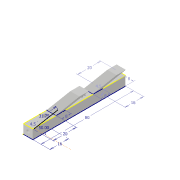
# Autodesk Inventor part: MineralStop1.25x50
Saved by Autodesk Inventor 2018 (Build 220112000, 112)
## iProperties
Created: 2018-12-12
Part Number: MineralStop1.25x50
Material: Generic
Document SubType Name: Modeling
Designer: ball
Density: 1 g/cm^3
Appearance: Default
Author: ball
Autodesk Inventor part; units mm, degrees
ref_plane "YZ Plane" through (0, 0, 0) normal (1, 0, 0) x (0, 1, 0)
ref_plane "XZ Plane" through (0, 0, 0) normal (0, 1, 0) x (-1, 0, 0)
ref_plane "XY Plane" through (0, 0, 0) normal (0, 0, 1) x (1, 0, 0)
sketch "Sketch1" plane through (0, 0, 0) normal (0, 1, 0) x (-1, 0, 0)
  line L0 (0, 0) -> (-8, 0)
  line L1 (-8, 0) -> (-8, -80)
  line L2 (-8, -80) -> (0, -80)
  line L3 (0, -80) -> (0, 0)
  circle A0 centre (-4, -16) radius 2.25
  circle A1 centre (-4, -64) radius 2.25
  dimension "d0" = 8
  dimension "d1" = 80
  dimension "d6" = 4.5
  dimension "d7" = 4.5
  dimension "d26" = 16
  dimension "d27" = 16
  constraints: 8 end point, 2 centre point, 2 parallel, 1 horizontal, 1 perpendicular
  measures "d0" distance of L2.end L1.end
  measures "d1" distance of L1.end L0.end
  measures "d6" diameter of A0
  measures "d7" diameter of A1
  measures "d26" distance from line of L0 A0.centre
  measures "d27" distance from line of L2 A1.centre
extrude "Extrusion1" [suppressed]
extrude "Extrusion2" add sketch "Sketch1" along normal blind 8
sketch "Sketch2" plane through (0, 0, 0) normal (0, 0, 1) x (1, 0, 0)
  circle A0 centre (4, 4) radius 1.35
  point P0 (0, 0)
  dimension "d10" = 2.7
  constraints: 1 centre point
  measures "d10" diameter of A0
hole "Hole1" at (4, 4, 0) direction (0, 0, -1) diameter 2.7 depth 10
sketch "Sketch3" plane through (8, 0, -80) normal (0, 0, -1) x (-1, 0, 0)
  circle A0 centre (4, 4) radius 1.35
  point P0 (8, 0)
  dimension "d18" = 2.7
  constraints: 1 centre point
  measures "d18" diameter of A0
hole "Hole2" at (4, 4, -80) direction (0, 0, 1) diameter 2.7 depth 10
sketch "Sketch5" plane through (0, 0, 0) normal (0, 0, 1) x (1, 0, 0)
  line L0 (9.3659, 8.9784) -> (29.7744, 33.3003)
  line L1 (9.3659, 8.9784) -> (41.1159, 8.9784) construction
  point P0 (0, 0)
  dimension "d33" = 31.75
  dimension "d34" = 50
  constraints: 4 end point, 1 equal length, 1 horizontal
  measures "d33" distance of L0.start L0.end
  measures "d34" angle of L1 L0
sketch "Sketch4" plane through (0, 8, 0) normal (0, 1, 0) x (1, 0, 0)
  line L0 (0, 80) -> (0, 0) projected
  line L1 (8, 0) -> (8, 80) projected
  line L2 (0, 28) -> (8, 28)
  line L3 (8, 28) -> (8, 20)
  line L4 (8, 20) -> (0, 20)
  line L5 (0, 20) -> (0, 28)
  line L6 (0, 0) -> (8, 0) projected
  line L7 (0, 60) -> (8, 60)
  line L8 (8, 60) -> (8, 52)
  line L9 (8, 52) -> (0, 52)
  line L10 (0, 52) -> (0, 60)
  line L11 (8, 80) -> (0, 80) projected
  line L12 (2.6299, 29.4213) -> (2.6299, 50.4758) construction
  line L13 (2.6299, 50.4758) -> (5.8779, 50.4758) construction
  line L14 (5.8779, 50.4758) -> (5.8779, 29.4213) construction
  line L15 (5.8779, 29.4213) -> (2.6299, 29.4213) construction
  line L16 (5.8137, 31.3702) -> (5.8137, 29.8832)
  line L17 (5.8137, 29.8832) -> (5.5025, 29.8832)
  line L18 (5.5025, 29.8832) -> (5.5025, 30.4365)
  line L19 (5.5025, 30.4365) -> (3.4598, 30.4365)
  line L20 (3.4598, 30.4365) -> (3.4598, 29.8832)
  line L21 (3.4598, 29.8832) -> (3.1807, 29.8832)
  spline S0 degree 2 poles (3.1807, 29.8832) (3.1807, 30.1969) (3.0028, 30.4933) (2.7558, 30.5131) knots 0 0 0 1 2 2 2
  line L22 (2.7558, 30.5131) -> (2.7558, 30.8292)
  line L23 (2.7558, 30.8292) -> (5.5025, 30.8292)
  line L24 (5.5025, 30.8292) -> (5.5025, 31.3702)
  line L25 (5.5025, 31.3702) -> (5.8137, 31.3702)
  line L26 (5.8137, 32.5854) -> (5.8137, 32.0964)
  line L27 (5.8137, 32.0964) -> (5.2308, 32.0964)
  line L28 (5.2308, 32.0964) -> (5.2308, 32.5854)
  line L29 (5.2308, 32.5854) -> (5.8137, 32.5854)
  line L30 (5.8137, 35.0801) -> (5.8137, 33.2005)
  line L31 (5.8137, 33.2005) -> (5.3815, 33.2005)
  spline S1 degree 2 poles (5.3815, 33.2005) (5.1913, 33.403) (4.838, 33.7636) (4.6479, 33.9365) knots 0 0 0 1 2 2 2
  spline S2 degree 2 poles (4.6479, 33.9365) (4.265, 34.2848) (3.8056, 34.5392) (3.561, 34.5392) knots 0 0 0 1 2 2 2
  spline S3 degree 2 poles (3.561, 34.5392) (3.4326, 34.5392) (3.2399, 34.4602) (3.1782, 34.3885) knots 0 0 0 1 2 2 2
  spline S4 degree 2 poles (3.1782, 34.3885) (3.1164, 34.3169) (3.0547, 34.1292) (3.0547, 34.0156) knots 0 0 0 1 2 2 2
  spline S5 degree 2 poles (3.0547, 34.0156) (3.0547, 33.9069) (3.109, 33.6846) (3.151, 33.5833) knots 0 0 0 1 2 2 2
  spline S6 degree 2 poles (3.151, 33.5833) (3.1856, 33.4969) (3.2844, 33.3363) (3.319, 33.2869) knots 0 0 0 1 2 2 2
  line L32 (3.319, 33.2869) -> (3.319, 33.2647)
  line L33 (3.319, 33.2647) -> (2.8843, 33.2647)
  spline S7 degree 2 poles (2.8843, 33.2647) (2.8225, 33.3907) (2.7015, 33.8427) (2.7015, 34.0452) knots 0 0 0 1 2 2 2
  spline S8 degree 2 poles (2.7015, 34.0452) (2.7015, 34.4725) (3.1535, 34.9542) (3.5388, 34.9542) knots 0 0 0 1 2 2 2
  spline S9 degree 2 poles (3.5388, 34.9542) (3.7191, 34.9542) (4.0205, 34.8702) (4.1489, 34.7961) knots 0 0 0 1 2 2 2
  spline S10 degree 2 poles (4.1489, 34.7961) (4.2823, 34.722) (4.5441, 34.5071) (4.6701, 34.3885) knots 0 0 0 1 2 2 2
  spline S11 degree 2 poles (4.6701, 34.3885) (4.88, 34.1959) (5.3296, 33.7241) (5.4605, 33.5833) knots 0 0 0 1 2 2 2
  line L34 (5.4605, 33.5833) -> (5.4605, 35.0801)
  line L35 (5.4605, 35.0801) -> (5.8137, 35.0801)
  spline S12 degree 2 poles (4.8455, 37.3353) (5.0653, 37.3353) (5.4407, 37.1945) (5.5791, 37.066) knots 0 0 0 1 2 2 2
  spline S13 degree 2 poles (5.5791, 37.066) (5.7174, 36.9376) (5.8779, 36.5547) (5.8779, 36.3176) knots 0 0 0 1 2 2 2
  spline S14 degree 2 poles (5.8779, 36.3176) (5.8779, 36.1003) (5.7816, 35.6754) (5.705, 35.5198) knots 0 0 0 1 2 2 2
  line L36 (5.705, 35.5198) -> (5.2728, 35.5198)
  line L37 (5.2728, 35.5198) -> (5.2728, 35.5494)
  spline S15 degree 2 poles (5.2728, 35.5494) (5.3074, 35.5964) (5.3963, 35.7717) (5.4358, 35.878) knots 0 0 0 1 2 2 2
  spline S16 degree 2 poles (5.4358, 35.878) (5.4778, 35.999) (5.5247, 36.1991) (5.5247, 36.325) knots 0 0 0 1 2 2 2
  spline S17 degree 2 poles (5.5247, 36.325) (5.5247, 36.4485) (5.4358, 36.6807) (5.3395, 36.7647) knots 0 0 0 1 2 2 2
  spline S18 degree 2 poles (5.3395, 36.7647) (5.2481, 36.8413) (5.006, 36.9203) (4.843, 36.9203) knots 0 0 0 1 2 2 2
  spline S19 degree 2 poles (4.843, 36.9203) (4.68, 36.9203) (4.4725, 36.8314) (4.4033, 36.7474) knots 0 0 0 1 2 2 2
  spline S20 degree 2 poles (4.4033, 36.7474) (4.3268, 36.661) (4.2625, 36.4041) (4.2625, 36.2485) knots 0 0 0 1 2 2 2
  spline S21 degree 2 poles (4.2625, 36.2485) (4.2625, 36.0805) (4.3144, 35.747) (4.3366, 35.6458) knots 0 0 0 1 2 2 2
  line L38 (4.3366, 35.6458) -> (2.7657, 35.6458)
  line L39 (2.7657, 35.6458) -> (2.7657, 37.318)
  line L40 (2.7657, 37.318) -> (3.1239, 37.318)
  line L41 (3.1239, 37.318) -> (3.1239, 36.0385)
  line L42 (3.1239, 36.0385) -> (3.9365, 36.0385)
  spline S22 degree 2 poles (3.9365, 36.0385) (3.9266, 36.1126) (3.9192, 36.2559) (3.9192, 36.3152) knots 0 0 0 1 2 2 2
  spline S23 degree 2 poles (3.9192, 36.3152) (3.9192, 36.5498) (3.9958, 36.8734) (4.1094, 37.0216) knots 0 0 0 1 2 2 2
  spline S24 degree 2 poles (4.1094, 37.0216) (4.223, 37.1722) (4.5688, 37.3353) (4.8455, 37.3353) knots 0 0 0 1 2 2 2
  line L43 (2.6299, 38.2319) -> (3.8155, 38.143)
  line L44 (3.8155, 38.143) -> (3.8155, 37.8737)
  line L45 (3.8155, 37.8737) -> (2.6299, 37.7848)
  line L46 (2.6299, 37.7848) -> (2.6299, 38.2319)
  line L47 (2.6299, 39.0025) -> (3.8155, 38.9136)
  line L48 (3.8155, 38.9136) -> (3.8155, 38.6444)
  line L49 (3.8155, 38.6444) -> (2.6299, 38.5555)
  line L50 (2.6299, 38.5555) -> (2.6299, 39.0025)
  line L51 (5.8137, 42.5989) -> (5.8137, 42.1271)
  line L52 (5.8137, 42.1271) -> (4.9541, 41.5713)
  line L53 (4.9541, 41.5713) -> (5.8137, 41.0008)
  line L54 (5.8137, 41.0008) -> (5.8137, 40.5636)
  line L55 (5.8137, 40.5636) -> (4.68, 41.3565)
  line L56 (4.68, 41.3565) -> (3.5265, 40.571)
  line L57 (3.5265, 40.571) -> (3.5265, 41.0428)
  line L58 (3.5265, 41.0428) -> (4.3786, 41.596)
  line L59 (4.3786, 41.596) -> (3.5265, 42.1617)
  line L60 (3.5265, 42.1617) -> (3.5265, 42.5989)
  line L61 (3.5265, 42.5989) -> (4.6553, 41.8109)
  line L62 (4.6553, 41.8109) -> (5.8137, 42.5989)
  spline S25 degree 2 poles (4.8455, 45.9976) (5.0653, 45.9976) (5.4407, 45.8568) (5.5791, 45.7284) knots 0 0 0 1 2 2 2
  spline S26 degree 2 poles (5.5791, 45.7284) (5.7174, 45.5999) (5.8779, 45.2171) (5.8779, 44.98) knots 0 0 0 1 2 2 2
  spline S27 degree 2 poles (5.8779, 44.98) (5.8779, 44.7626) (5.7816, 44.3378) (5.705, 44.1822) knots 0 0 0 1 2 2 2
  line L63 (5.705, 44.1822) -> (5.2728, 44.1822)
  line L64 (5.2728, 44.1822) -> (5.2728, 44.2118)
  spline S28 degree 2 poles (5.2728, 44.2118) (5.3074, 44.2587) (5.3963, 44.4341) (5.4358, 44.5403) knots 0 0 0 1 2 2 2
  spline S29 degree 2 poles (5.4358, 44.5403) (5.4778, 44.6613) (5.5247, 44.8614) (5.5247, 44.9874) knots 0 0 0 1 2 2 2
  spline S30 degree 2 poles (5.5247, 44.9874) (5.5247, 45.1109) (5.4358, 45.3431) (5.3395, 45.427) knots 0 0 0 1 2 2 2
  spline S31 degree 2 poles (5.3395, 45.427) (5.2481, 45.5036) (5.006, 45.5827) (4.843, 45.5827) knots 0 0 0 1 2 2 2
  spline S32 degree 2 poles (4.843, 45.5827) (4.68, 45.5827) (4.4725, 45.4937) (4.4033, 45.4098) knots 0 0 0 1 2 2 2
  spline S33 degree 2 poles (4.4033, 45.4098) (4.3268, 45.3233) (4.2625, 45.0664) (4.2625, 44.9108) knots 0 0 0 1 2 2 2
  spline S34 degree 2 poles (4.2625, 44.9108) (4.2625, 44.7428) (4.3144, 44.4094) (4.3366, 44.3081) knots 0 0 0 1 2 2 2
  line L65 (4.3366, 44.3081) -> (2.7657, 44.3081)
  line L66 (2.7657, 44.3081) -> (2.7657, 45.9803)
  line L67 (2.7657, 45.9803) -> (3.1239, 45.9803)
  line L68 (3.1239, 45.9803) -> (3.1239, 44.7009)
  line L69 (3.1239, 44.7009) -> (3.9365, 44.7009)
  spline S35 degree 2 poles (3.9365, 44.7009) (3.9266, 44.775) (3.9192, 44.9182) (3.9192, 44.9775) knots 0 0 0 1 2 2 2
  spline S36 degree 2 poles (3.9192, 44.9775) (3.9192, 45.2121) (3.9958, 45.5357) (4.1094, 45.6839) knots 0 0 0 1 2 2 2
  spline S37 degree 2 poles (4.1094, 45.6839) (4.223, 45.8346) (4.5688, 45.9976) (4.8455, 45.9976) knots 0 0 0 1 2 2 2
  spline S38 degree 2 poles (4.2897, 48.3342) (5.1097, 48.3342) (5.8779, 47.8575) (5.8779, 47.3611) knots 0 0 0 1 2 2 2
  spline S39 degree 2 poles (5.8779, 47.3611) (5.8779, 46.8572) (5.0949, 46.3854) (4.2922, 46.3854) knots 0 0 0 1 2 2 2
  spline S40 degree 2 poles (4.2922, 46.3854) (3.4672, 46.3854) (2.704, 46.8621) (2.704, 47.3611) knots 0 0 0 1 2 2 2
  spline S41 degree 2 poles (2.704, 47.3611) (2.704, 47.8625) (3.4944, 48.3342) (4.2897, 48.3342) knots 0 0 0 1 2 2 2
  spline S42 degree 2 poles (5.2184, 47.8106) (5.0678, 47.8699) (4.6034, 47.9193) (4.2897, 47.9193) knots 0 0 0 1 2 2 2
  spline S43 degree 2 poles (4.2897, 47.9193) (3.976, 47.9193) (3.5141, 47.8699) (3.3585, 47.8081) knots 0 0 0 1 2 2 2
  spline S44 degree 2 poles (3.3585, 47.8081) (3.2029, 47.7464) (3.0423, 47.5315) (3.0423, 47.3611) knots 0 0 0 1 2 2 2
  spline S45 degree 2 poles (3.0423, 47.3611) (3.0423, 47.1906) (3.2029, 46.9708) (3.3634, 46.9066) knots 0 0 0 1 2 2 2
  spline S46 degree 2 poles (3.3634, 46.9066) (3.5191, 46.8448) (3.9933, 46.8004) (4.2922, 46.8004) knots 0 0 0 1 2 2 2
  spline S47 degree 2 poles (4.2922, 46.8004) (4.6133, 46.8004) (5.0431, 46.8399) (5.211, 46.9041) knots 0 0 0 1 2 2 2
  spline S48 degree 2 poles (5.211, 46.9041) (5.3691, 46.9634) (5.5395, 47.1832) (5.5395, 47.3611) knots 0 0 0 1 2 2 2
  spline S49 degree 2 poles (5.5395, 47.3611) (5.5395, 47.529) (5.379, 47.7489) (5.2184, 47.8106) knots 0 0 0 1 2 2 2
  spline S50 degree 2 poles (3.4919, 50.2683) (3.8204, 50.2683) (4.2699, 49.8187) (4.2699, 49.4902) knots 0 0 0 1 2 2 2
  spline S51 degree 2 poles (4.2699, 49.4902) (4.2699, 49.1642) (3.8229, 48.7097) (3.4919, 48.7097) knots 0 0 0 1 2 2 2
  spline S52 degree 2 poles (3.4919, 48.7097) (3.1634, 48.7097) (2.7138, 49.1592) (2.7138, 49.4902) knots 0 0 0 1 2 2 2
  spline S53 degree 2 poles (2.7138, 49.4902) (2.7138, 49.8187) (3.1634, 50.2683) (3.4919, 50.2683) knots 0 0 0 1 2 2 2
  spline S54 degree 2 poles (3.4919, 49.9472) (3.2943, 49.9472) (3.0251, 49.6853) (3.0251, 49.4902) knots 0 0 0 1 2 2 2
  spline S55 degree 2 poles (3.0251, 49.4902) (3.0251, 49.2926) (3.2943, 49.0308) (3.4919, 49.0308) knots 0 0 0 1 2 2 2
  spline S56 degree 2 poles (3.4919, 49.0308) (3.692, 49.0308) (3.9587, 49.2976) (3.9587, 49.4902) knots 0 0 0 1 2 2 2
  spline S57 degree 2 poles (3.9587, 49.4902) (3.9587, 49.6853) (3.687, 49.9472) (3.4919, 49.9472) knots 0 0 0 1 2 2 2
  dimension "d28" = 8
  dimension "d29" = 20
  dimension "d30" = 8
  dimension "d31" = 20
  constraints: 16 end point, 4 parallel, 4 point on line, 2 horizontal, 2 perpendicular, 2 other
  measures "d28" distance of L2.end L3.end
  measures "d29" distance between parallel lines of L6 L4
  measures "d30" distance of L7.end L8.end
  measures "d31" distance between parallel lines of L11 L7
sweep "Sweep1" add profiles "Sketch4" path "Sketch5" contours L2 L1 L4 L0
sweep "Sweep2" add profiles "Sketch4" path "Sketch5" contours L7 L1 L9 L0
emboss "Emboss1" sketch "Sketch4" operation add depth 1 direction (0, -1, 0) contours L16 L17 L18 L19 L20 L21 S0 L22 L23 L24 L25 | L26 L27 L28 L29 | L30 L31 S1 S2 S3 S4 S5 S6 L32 L33 S7 S8 S9 S10 S11 L34 L35 | S12 S13 S14 L36 L37 S15 S16 S17 S18 S19 S20 S21 L38 L39 L40 L41 L42 S22 S23 S24 | L43 L44 L45 L46 | L47 L48 L49 L50 | L51 L52 L53 L54 L55 L56 L57 L58 L59 L60 L61 L62 | S25 S26 S27 L63 L64 S28 S29 S30 S31 S32 S33 S34 L65 L66 L67 L68 L69 S35 S36 S37 | S38 S39 S40 S41 | S50 S51 S52 S53
body "Solid1"
